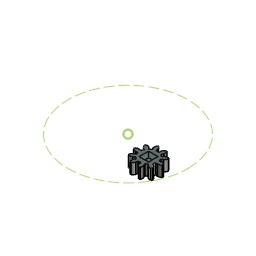
Electronics box (Autodesk Fusion 360 archive; units mm, degrees)
design "small gear"
description: Spur Gear; Module: 12.7; Num Teeth: 10; Pressure Angle: 20.0; Backlash: 0.00 mm
Autodesk Fusion 360 part; units mm, degrees
(part 1 of 4)
sketch "Sketch1" plane through (0, 0, 0) normal (0, 0, 1) x (1, 0, 0) in component "Spur Gear (10 teeth)"
  circle A0 centre (0, 0) radius 48.2092
  circle A1 centre (0, 0) radius 6.35
extrude "Extrude1" add sketch "Sketch1" along normal blind 12.7 in component "Spur Gear (10 teeth)"
sketch "Sketch2" plane through (0, 0, 0) normal (0, 0, 1) x (1, 0, 0) in component "Spur Gear (10 teeth)"
  spline S0 degree 5 poles (58.7902, -10.2119) (58.8398, -10.2205) (58.9391, -10.2359) (59.0886, -10.2539) (59.2889, -10.2679) (59.5405, -10.2721) (59.7929, -10.2667) (60.0458, -10.2556) (60.2991, -10.2415) (60.5524, -10.2252) (60.8059, -10.2064) (61.0595, -10.1843) (61.3132, -10.158) (61.5672, -10.1267) (61.8213, -10.0907) (62.0755, -10.0504) (62.3297, -10.0065) (62.5839, -9.9595) (62.838, -9.9098) (63.092, -9.8574) (63.3459, -9.8024) (63.5998, -9.7445) (63.8535, -9.6836) (64.107, -9.6197) (64.3605, -9.5529) (64.6138, -9.4832) (64.8669, -9.4108) (65.1198, -9.3359) (65.3724, -9.2586) (65.6249, -9.1787) (65.8771, -9.0965) (66.129, -9.0118) (66.3807, -8.9247) (66.6321, -8.8352) (66.8832, -8.7433) (67.134, -8.649) (67.3844, -8.5525) (67.6346, -8.4537) (67.8844, -8.3527) (68.1338, -8.2495) (68.3829, -8.1441) (68.6317, -8.0366) (68.88, -7.9269) (69.128, -7.8151) (69.3755, -7.7012) (69.6227, -7.5852) (69.8694, -7.4672) (70.1157, -7.3471) (70.3615, -7.2251) (70.6069, -7.101) (70.8519, -6.9749) (71.0964, -6.8469) (71.3404, -6.7169) (71.5839, -6.5851) (71.827, -6.4512) (72.0695, -6.3155) (72.3115, -6.1779) (72.5531, -6.0384) (72.7941, -5.8971) (73.0345, -5.7539) (73.2744, -5.6089) (73.5138, -5.4621) (73.7527, -5.3135) (73.9909, -5.1631) (74.2286, -5.0109) (74.4657, -4.857) (74.7023, -4.7013) (74.9382, -4.5438) (75.1735, -4.3847) (75.4083, -4.2238) (75.6424, -4.0612) (75.8292, -3.9298) (75.969, -3.8304) (76.0621, -3.7639) (76.1086, -3.7305) knots 0 0 0 0 0 0 0.01428571 0.02857143 0.04285714 0.05714286 0.07142857 0.08571429 0.1 0.11428571 0.12857143 0.14285714 0.15714286 0.17142857 0.18571429 0.2 0.21428571 0.22857143 0.24285714 0.25714286 0.27142857 0.28571429 0.3 0.31428571 0.32857143 0.34285714 0.35714286 0.37142857 0.38571429 0.4 0.41428571 0.42857143 0.44285714 0.45714286 0.47142857 0.48571429 0.5 0.51428571 0.52857143 0.54285714 0.55714286 0.57142857 0.58571429 0.6 0.61428571 0.62857143 0.64285714 0.65714286 0.67142857 0.68571429 0.7 0.71428571 0.72857143 0.74285714 0.75714286 0.77142857 0.78571429 0.8 0.81428571 0.82857143 0.84285714 0.85714286 0.87142857 0.88571429 0.9 0.91428571 0.92857143 0.94285714 0.95714286 0.97142857 0.98571429 1 1 1 1 1 1
  spline S1 degree 5 poles (58.7902, 10.2119) (58.8398, 10.2205) (58.9391, 10.2359) (59.0886, 10.2539) (59.2889, 10.2679) (59.5405, 10.2721) (59.7929, 10.2667) (60.0458, 10.2556) (60.2991, 10.2415) (60.5524, 10.2252) (60.8059, 10.2064) (61.0595, 10.1843) (61.3132, 10.158) (61.5672, 10.1267) (61.8213, 10.0907) (62.0755, 10.0504) (62.3297, 10.0065) (62.5839, 9.9595) (62.838, 9.9098) (63.092, 9.8574) (63.3459, 9.8024) (63.5998, 9.7445) (63.8535, 9.6836) (64.107, 9.6197) (64.3605, 9.5529) (64.6138, 9.4832) (64.8669, 9.4108) (65.1198, 9.3359) (65.3724, 9.2586) (65.6249, 9.1787) (65.8771, 9.0965) (66.129, 9.0118) (66.3807, 8.9247) (66.6321, 8.8352) (66.8832, 8.7433) (67.134, 8.649) (67.3844, 8.5525) (67.6346, 8.4537) (67.8844, 8.3527) (68.1338, 8.2495) (68.3829, 8.1441) (68.6317, 8.0366) (68.88, 7.9269) (69.128, 7.8151) (69.3755, 7.7012) (69.6227, 7.5852) (69.8694, 7.4672) (70.1157, 7.3471) (70.3615, 7.2251) (70.6069, 7.101) (70.8519, 6.9749) (71.0964, 6.8469) (71.3404, 6.7169) (71.5839, 6.5851) (71.827, 6.4512) (72.0695, 6.3155) (72.3115, 6.1779) (72.5531, 6.0384) (72.7941, 5.8971) (73.0345, 5.7539) (73.2744, 5.6089) (73.5138, 5.4621) (73.7527, 5.3135) (73.9909, 5.1631) (74.2286, 5.0109) (74.4657, 4.857) (74.7023, 4.7013) (74.9382, 4.5438) (75.1735, 4.3847) (75.4083, 4.2238) (75.6424, 4.0612) (75.8292, 3.9298) (75.969, 3.8304) (76.0621, 3.7639) (76.1086, 3.7305) knots 0 0 0 0 0 0 0.01428571 0.02857143 0.04285714 0.05714286 0.07142857 0.08571429 0.1 0.11428571 0.12857143 0.14285714 0.15714286 0.17142857 0.18571429 0.2 0.21428571 0.22857143 0.24285714 0.25714286 0.27142857 0.28571429 0.3 0.31428571 0.32857143 0.34285714 0.35714286 0.37142857 0.38571429 0.4 0.41428571 0.42857143 0.44285714 0.45714286 0.47142857 0.48571429 0.5 0.51428571 0.52857143 0.54285714 0.55714286 0.57142857 0.58571429 0.6 0.61428571 0.62857143 0.64285714 0.65714286 0.67142857 0.68571429 0.7 0.71428571 0.72857143 0.74285714 0.75714286 0.77142857 0.78571429 0.8 0.81428571 0.82857143 0.84285714 0.85714286 0.87142857 0.88571429 0.9 0.91428571 0.92857143 0.94285714 0.95714286 0.97142857 0.98571429 1 1 1 1 1 1
  arc A0 (76.1086, -3.7305) -> (76.1086, 3.7305) centre (0, 0) ccw
  line L0 (47.4881, -8.2504) -> (58.7902, -10.2119)
  line L1 (47.4881, 8.2504) -> (58.7902, 10.2119)
  line L2 (47.4881, -8.2504) -> (47.4881, 8.2504)
  point P0 (59.9803, -10.2579)
  point P1 (61.1925, -10.1699)
  point P2 (62.4182, -9.9897)
  point P3 (63.6537, -9.7311)
  point P4 (64.8964, -9.4016)
  point P5 (66.1443, -9.006)
  point P6 (67.3954, -8.5476)
  point P7 (68.648, -8.0288)
  point P8 (69.9005, -7.4516)
  point P9 (71.1514, -6.8172)
  point P10 (72.3992, -6.127)
  point P11 (73.6422, -5.382)
  point P12 (74.8792, -4.5829)
  point P13 (59.9803, 10.2579)
  point P14 (61.1925, 10.1699)
  point P15 (62.4182, 9.9897)
  point P16 (63.6537, 9.7311)
  point P17 (64.8964, 9.4016)
  point P18 (66.1443, 9.006)
  point P19 (67.3954, 8.5476)
  point P20 (68.648, 8.0288)
  point P21 (69.9005, 7.4516)
  point P22 (71.1514, 6.8172)
  point P23 (72.3992, 6.127)
  point P24 (73.6422, 5.382)
  point P25 (74.8792, 4.5829)
extrude "Extrude2" add sketch "Sketch2" along normal blind 12.7 in component "Spur Gear (10 teeth)"
fillet "Fillet1" radius 1.5875 2 edges at (47.4977, -8.2521, 6.35) (47.4977, 8.2521, 6.35) in component "Spur Gear (10 teeth)"
pattern_circular "C-Pattern1" count 10 over 360 about axis through (0, 0, 0) along (0, 0, 1) of "Extrude2", "Fillet1" in component "Spur Gear (10 teeth)"
sketch "Sketch3" plane through (0, 0, 0) normal (0, 0, 1) x (1, 0, 0) in component "Spur Gear (10 teeth)"
  circle A0 centre (0, 0) radius 63.5 construction
scale "Scale1" factor 0.2 about (53.5646, -26.2944, 0) bodies 1 in component "Spur Gear (10 teeth)"
extrude "Extrude3" add 1 faces at (37.4307, -25.0246, 2.54) along direction (0, 0, 1) blind 8.73 in component "Spur Gear (10 teeth)"
sketch "Sketch2 (2)" plane through (0, 0, 11.27) normal (0, 0, 1) x (-1, 0, 0)
  arc A0 (-51.6381, 25.006) -> (-52.2938, 22.9879) centre (-42.8517, 21.0355) ccw
  arc A1 (-52.659, 22.7394) -> (-52.2938, 22.9879) centre (-52.6047, 23.0522) ccw
  line L0 (-52.659, 22.7394) -> (-54.6097, 23.0779)
  spline S0 degree 5 poles (-54.6097, 23.0779) (-54.6197, 23.0796) (-54.6395, 23.0827) (-54.6694, 23.0863) (-54.7095, 23.0891) (-54.7598, 23.09) (-54.8103, 23.0889) (-54.8609, 23.0867) (-54.9115, 23.0838) (-54.9622, 23.0806) (-55.0129, 23.0768) (-55.0636, 23.0724) (-55.1143, 23.0671) (-55.1651, 23.0609) (-55.216, 23.0537) (-55.2668, 23.0456) (-55.3176, 23.0368) (-55.3685, 23.0274) (-55.4193, 23.0175) (-55.4701, 23.007) (-55.5209, 22.996) (-55.5717, 22.9844) (-55.6224, 22.9723) (-55.6731, 22.9595) (-55.7238, 22.9461) (-55.7745, 22.9322) (-55.8251, 22.9177) (-55.8757, 22.9027) (-55.9262, 22.8873) (-55.9767, 22.8713) (-56.0271, 22.8548) (-56.0775, 22.8379) (-56.1278, 22.8205) (-56.1781, 22.8026) (-56.2283, 22.7842) (-56.2785, 22.7653) (-56.3286, 22.746) (-56.3786, 22.7263) (-56.4286, 22.7061) (-56.4785, 22.6854) (-56.5283, 22.6644) (-56.578, 22.6429) (-56.6277, 22.6209) (-56.6773, 22.5986) (-56.7268, 22.5758) (-56.7762, 22.5526) (-56.8256, 22.529) (-56.8748, 22.505) (-56.924, 22.4806) (-56.9731, 22.4557) (-57.0221, 22.4305) (-57.071, 22.4049) (-57.1198, 22.3789) (-57.1685, 22.3526) (-57.2171, 22.3258) (-57.2656, 22.2987) (-57.314, 22.2711) (-57.3623, 22.2432) (-57.4105, 22.215) (-57.4586, 22.1863) (-57.5066, 22.1573) (-57.5545, 22.128) (-57.6022, 22.0982) (-57.6499, 22.0682) (-57.6974, 22.0377) (-57.7448, 22.0069) (-57.7922, 21.9758) (-57.8393, 21.9443) (-57.8864, 21.9125) (-57.9334, 21.8803) (-57.9802, 21.8478) (-58.0175, 21.8215) (-58.0455, 21.8016) (-58.0641, 21.7883) (-58.0734, 21.7816) knots 0 0 0 0 0 0 0.01428571 0.02857143 0.04285714 0.05714286 0.07142857 0.08571429 0.1 0.11428571 0.12857143 0.14285714 0.15714286 0.17142857 0.18571429 0.2 0.21428571 0.22857143 0.24285714 0.25714286 0.27142857 0.28571429 0.3 0.31428571 0.32857143 0.34285714 0.35714286 0.37142857 0.38571429 0.4 0.41428571 0.42857143 0.44285714 0.45714286 0.47142857 0.48571429 0.5 0.51428571 0.52857143 0.54285714 0.55714286 0.57142857 0.58571429 0.6 0.61428571 0.62857143 0.64285714 0.65714286 0.67142857 0.68571429 0.7 0.71428571 0.72857143 0.74285714 0.75714286 0.77142857 0.78571429 0.8 0.81428571 0.82857143 0.84285714 0.85714286 0.87142857 0.88571429 0.9 0.91428571 0.92857143 0.94285714 0.95714286 0.97142857 0.98571429 1 1 1 1 1 1
  arc A2 (-58.0734, 21.7816) -> (-58.0734, 20.2895) centre (-42.8517, 21.0355) ccw
  spline S1 degree 5 poles (-58.0734, 20.2895) (-58.0641, 20.2828) (-58.0455, 20.2695) (-58.0175, 20.2496) (-57.9802, 20.2233) (-57.9334, 20.1908) (-57.8864, 20.1586) (-57.8393, 20.1268) (-57.7922, 20.0953) (-57.7448, 20.0642) (-57.6974, 20.0334) (-57.6499, 20.0029) (-57.6022, 19.9728) (-57.5545, 19.9431) (-57.5066, 19.9138) (-57.4586, 19.8848) (-57.4105, 19.8561) (-57.3623, 19.8279) (-57.314, 19.8) (-57.2656, 19.7724) (-57.2171, 19.7453) (-57.1685, 19.7185) (-57.1198, 19.6922) (-57.071, 19.6662) (-57.0221, 19.6406) (-56.9731, 19.6154) (-56.924, 19.5905) (-56.8748, 19.5661) (-56.8256, 19.5421) (-56.7762, 19.5185) (-56.7268, 19.4953) (-56.6773, 19.4725) (-56.6277, 19.4502) (-56.578, 19.4282) (-56.5283, 19.4067) (-56.4785, 19.3857) (-56.4286, 19.365) (-56.3786, 19.3448) (-56.3286, 19.3251) (-56.2785, 19.3057) (-56.2283, 19.2869) (-56.1781, 19.2685) (-56.1278, 19.2506) (-56.0775, 19.2332) (-56.0271, 19.2162) (-55.9767, 19.1998) (-55.9262, 19.1838) (-55.8757, 19.1684) (-55.8251, 19.1534) (-55.7745, 19.1389) (-55.7238, 19.125) (-55.6731, 19.1116) (-55.6224, 19.0988) (-55.5717, 19.0866) (-55.5209, 19.0751) (-55.4701, 19.0641) (-55.4193, 19.0536) (-55.3685, 19.0437) (-55.3176, 19.0343) (-55.2668, 19.0255) (-55.216, 19.0174) (-55.1651, 19.0102) (-55.1143, 19.004) (-55.0636, 18.9987) (-55.0129, 18.9943) (-54.9622, 18.9905) (-54.9115, 18.9873) (-54.8609, 18.9844) (-54.8103, 18.9822) (-54.7598, 18.9811) (-54.7095, 18.982) (-54.6694, 18.9848) (-54.6395, 18.9884) (-54.6197, 18.9915) (-54.6097, 18.9932) knots -1 -1 -1 -1 -1 -1 -0.98571429 -0.97142857 -0.95714286 -0.94285714 -0.92857143 -0.91428571 -0.9 -0.88571429 -0.87142857 -0.85714286 -0.84285714 -0.82857143 -0.81428571 -0.8 -0.78571429 -0.77142857 -0.75714286 -0.74285714 -0.72857143 -0.71428571 -0.7 -0.68571429 -0.67142857 -0.65714286 -0.64285714 -0.62857143 -0.61428571 -0.6 -0.58571429 -0.57142857 -0.55714286 -0.54285714 -0.52857143 -0.51428571 -0.5 -0.48571429 -0.47142857 -0.45714286 -0.44285714 -0.42857143 -0.41428571 -0.4 -0.38571429 -0.37142857 -0.35714286 -0.34285714 -0.32857143 -0.31428571 -0.3 -0.28571429 -0.27142857 -0.25714286 -0.24285714 -0.22857143 -0.21428571 -0.2 -0.18571429 -0.17142857 -0.15714286 -0.14285714 -0.12857143 -0.11428571 -0.1 -0.08571429 -0.07142857 -0.05714286 -0.04285714 -0.02857143 -0.01428571 0 0 0 0 0 0
  line L1 (-54.6097, 18.9932) -> (-52.659, 19.3317)
  arc A3 (-52.2938, 19.0832) -> (-52.659, 19.3317) centre (-52.6047, 19.0189) ccw
  arc A4 (-52.2938, 19.0832) -> (-51.6381, 17.0651) centre (-42.8517, 21.0355) ccw
  arc A5 (-51.7875, 16.6494) -> (-51.6381, 17.0651) centre (-51.9274, 16.9344) ccw
  line L2 (-51.7875, 16.6494) -> (-53.5646, 15.7767)
  spline S2 degree 5 poles (-53.5646, 15.7767) (-53.5737, 15.7722) (-53.5916, 15.763) (-53.6179, 15.7484) (-53.6519, 15.7271) (-53.6931, 15.6982) (-53.7333, 15.6677) (-53.7729, 15.6361) (-53.8123, 15.6041) (-53.8513, 15.5716) (-53.8901, 15.5388) (-53.9286, 15.5054) (-53.9665, 15.4713) (-54.0039, 15.4364) (-54.0408, 15.4007) (-54.0772, 15.3643) (-54.1132, 15.3273) (-54.1488, 15.2898) (-54.1841, 15.2519) (-54.219, 15.2136) (-54.2536, 15.1748) (-54.2879, 15.1356) (-54.3218, 15.096) (-54.3553, 15.0558) (-54.3885, 15.0152) (-54.4212, 14.9742) (-54.4537, 14.9327) (-54.4858, 14.8908) (-54.5176, 14.8486) (-54.5491, 14.806) (-54.5802, 14.7631) (-54.611, 14.7198) (-54.6415, 14.6761) (-54.6716, 14.632) (-54.7015, 14.5876) (-54.731, 14.5429) (-54.7601, 14.4978) (-54.789, 14.4525) (-54.8175, 14.4067) (-54.8458, 14.3607) (-54.8737, 14.3144) (-54.9013, 14.2678) (-54.9286, 14.2208) (-54.9556, 14.1736) (-54.9822, 14.126) (-55.0086, 14.0782) (-55.0346, 14.0301) (-55.0604, 13.9817) (-55.0858, 13.9331) (-55.1109, 13.8842) (-55.1357, 13.835) (-55.1602, 13.7855) (-55.1844, 13.7358) (-55.2083, 13.6858) (-55.2319, 13.6356) (-55.2552, 13.5851) (-55.2782, 13.5344) (-55.3009, 13.4835) (-55.3233, 13.4323) (-55.3454, 13.3808) (-55.3671, 13.3292) (-55.3886, 13.2773) (-55.4098, 13.2251) (-55.4306, 13.1728) (-55.4512, 13.1202) (-55.4715, 13.0674) (-55.4914, 13.0144) (-55.5111, 12.9612) (-55.5305, 12.9078) (-55.5495, 12.8542) (-55.5683, 12.8004) (-55.5831, 12.7571) (-55.594, 12.7246) (-55.6013, 12.7029) (-55.6049, 12.692) knots 0 0 0 0 0 0 0.01428571 0.02857143 0.04285714 0.05714286 0.07142857 0.08571429 0.1 0.11428571 0.12857143 0.14285714 0.15714286 0.17142857 0.18571429 0.2 0.21428571 0.22857143 0.24285714 0.25714286 0.27142857 0.28571429 0.3 0.31428571 0.32857143 0.34285714 0.35714286 0.37142857 0.38571429 0.4 0.41428571 0.42857143 0.44285714 0.45714286 0.47142857 0.48571429 0.5 0.51428571 0.52857143 0.54285714 0.55714286 0.57142857 0.58571429 0.6 0.61428571 0.62857143 0.64285714 0.65714286 0.67142857 0.68571429 0.7 0.71428571 0.72857143 0.74285714 0.75714286 0.77142857 0.78571429 0.8 0.81428571 0.82857143 0.84285714 0.85714286 0.87142857 0.88571429 0.9 0.91428571 0.92857143 0.94285714 0.95714286 0.97142857 0.98571429 1 1 1 1 1 1
  arc A6 (-55.6049, 12.692) -> (-54.7278, 11.4848) centre (-42.8517, 21.0355) ccw
  spline S3 degree 5 poles (-54.7278, 11.4848) (-54.7163, 11.4849) (-54.6935, 11.4851) (-54.6591, 11.4854) (-54.6135, 11.4861) (-54.5565, 11.4874) (-54.4996, 11.4889) (-54.4428, 11.4908) (-54.3861, 11.4931) (-54.3295, 11.4957) (-54.2731, 11.4987) (-54.2167, 11.502) (-54.1605, 11.5057) (-54.1044, 11.5097) (-54.0484, 11.5141) (-53.9925, 11.5188) (-53.9368, 11.5239) (-53.8812, 11.5294) (-53.8257, 11.5352) (-53.7704, 11.5414) (-53.7152, 11.5479) (-53.6601, 11.5549) (-53.6052, 11.5622) (-53.5504, 11.5698) (-53.4958, 11.5778) (-53.4414, 11.5862) (-53.3871, 11.595) (-53.3329, 11.6042) (-53.279, 11.6137) (-53.2252, 11.6236) (-53.1716, 11.6339) (-53.1181, 11.6446) (-53.0649, 11.6556) (-53.0118, 11.6671) (-52.9589, 11.6789) (-52.9062, 11.6911) (-52.8537, 11.7038) (-52.8014, 11.7168) (-52.7493, 11.7302) (-52.6975, 11.744) (-52.6458, 11.7583) (-52.5944, 11.7729) (-52.5432, 11.788) (-52.4922, 11.8035) (-52.4415, 11.8194) (-52.391, 11.8357) (-52.3408, 11.8525) (-52.2908, 11.8697) (-52.2411, 11.8873) (-52.1916, 11.9053) (-52.1424, 11.9238) (-52.0936, 11.9428) (-52.045, 11.9623) (-51.9968, 11.9823) (-51.9489, 12.0027) (-51.9014, 12.0237) (-51.8541, 12.0451) (-51.8072, 12.0669) (-51.7605, 12.0892) (-51.7142, 12.1119) (-51.6684, 12.1353) (-51.623, 12.1594) (-51.5783, 12.1842) (-51.5341, 12.2097) (-51.4905, 12.236) (-51.4472, 12.2627) (-51.4043, 12.2899) (-51.3617, 12.3173) (-51.3195, 12.3453) (-51.278, 12.3741) (-51.2378, 12.4043) (-51.207, 12.4301) (-51.1849, 12.4506) (-51.1707, 12.4648) (-51.1637, 12.472) knots -1 -1 -1 -1 -1 -1 -0.98571429 -0.97142857 -0.95714286 -0.94285714 -0.92857143 -0.91428571 -0.9 -0.88571429 -0.87142857 -0.85714286 -0.84285714 -0.82857143 -0.81428571 -0.8 -0.78571429 -0.77142857 -0.75714286 -0.74285714 -0.72857143 -0.71428571 -0.7 -0.68571429 -0.67142857 -0.65714286 -0.64285714 -0.62857143 -0.61428571 -0.6 -0.58571429 -0.57142857 -0.55714286 -0.54285714 -0.52857143 -0.51428571 -0.5 -0.48571429 -0.47142857 -0.45714286 -0.44285714 -0.42857143 -0.41428571 -0.4 -0.38571429 -0.37142857 -0.35714286 -0.34285714 -0.32857143 -0.31428571 -0.3 -0.28571429 -0.27142857 -0.25714286 -0.24285714 -0.22857143 -0.21428571 -0.2 -0.18571429 -0.17142857 -0.15714286 -0.14285714 -0.12857143 -0.11428571 -0.1 -0.08571429 -0.07142857 -0.05714286 -0.04285714 -0.02857143 -0.01428571 0 0 0 0 0 0
  line L3 (-51.1637, 12.472) -> (-49.7845, 13.8925)
  arc A7 (-49.343, 13.9061) -> (-49.7845, 13.8925) centre (-49.5567, 13.6714) ccw
  arc A8 (-49.343, 13.9061) -> (-47.6263, 12.6589) centre (-42.8517, 21.0355) ccw
  arc A9 (-47.5028, 12.2347) -> (-47.6263, 12.6589) centre (-47.7835, 12.383) ccw
  line L4 (-47.5028, 12.2347) -> (-48.4275, 10.4841)
  spline S4 degree 5 poles (-48.4275, 10.4841) (-48.4322, 10.4752) (-48.4413, 10.4573) (-48.454, 10.4299) (-48.469, 10.3927) (-48.4854, 10.3451) (-48.4999, 10.2968) (-48.5135, 10.248) (-48.5264, 10.1989) (-48.539, 10.1497) (-48.5511, 10.1004) (-48.5626, 10.0508) (-48.5732, 10.0009) (-48.583, 9.9506) (-48.5918, 9.9001) (-48.5999, 9.8492) (-48.6072, 9.7982) (-48.614, 9.7469) (-48.6202, 9.6955) (-48.626, 9.644) (-48.6312, 9.5923) (-48.6359, 9.5404) (-48.64, 9.4884) (-48.6435, 9.4362) (-48.6465, 9.3839) (-48.6489, 9.3314) (-48.6507, 9.2788) (-48.6521, 9.226) (-48.653, 9.1732) (-48.6534, 9.1202) (-48.6534, 9.0672) (-48.6528, 9.014) (-48.6518, 8.9608) (-48.6503, 8.9074) (-48.6484, 8.854) (-48.6459, 8.8004) (-48.6431, 8.7468) (-48.6397, 8.6932) (-48.636, 8.6394) (-48.6317, 8.5856) (-48.6271, 8.5317) (-48.622, 8.4777) (-48.6165, 8.4237) (-48.6106, 8.3696) (-48.6042, 8.3155) (-48.5974, 8.2613) (-48.5902, 8.2071) (-48.5826, 8.1528) (-48.5746, 8.0985) (-48.5661, 8.0442) (-48.5573, 7.9898) (-48.5481, 7.9354) (-48.5384, 7.8809) (-48.5284, 7.8265) (-48.5179, 7.772) (-48.5071, 7.7174) (-48.4959, 7.6629) (-48.4843, 7.6083) (-48.4723, 7.5538) (-48.4599, 7.4992) (-48.4472, 7.4446) (-48.4341, 7.39) (-48.4206, 7.3354) (-48.4067, 7.2807) (-48.3924, 7.2261) (-48.3778, 7.1715) (-48.3628, 7.1169) (-48.3474, 7.0623) (-48.3317, 7.0077) (-48.3156, 6.9531) (-48.2991, 6.8985) (-48.2857, 6.8549) (-48.2754, 6.8221) (-48.2685, 6.8003) (-48.2651, 6.7894) knots 0 0 0 0 0 0 0.01428571 0.02857143 0.04285714 0.05714286 0.07142857 0.08571429 0.1 0.11428571 0.12857143 0.14285714 0.15714286 0.17142857 0.18571429 0.2 0.21428571 0.22857143 0.24285714 0.25714286 0.27142857 0.28571429 0.3 0.31428571 0.32857143 0.34285714 0.35714286 0.37142857 0.38571429 0.4 0.41428571 0.42857143 0.44285714 0.45714286 0.47142857 0.48571429 0.5 0.51428571 0.52857143 0.54285714 0.55714286 0.57142857 0.58571429 0.6 0.61428571 0.62857143 0.64285714 0.65714286 0.67142857 0.68571429 0.7 0.71428571 0.72857143 0.74285714 0.75714286 0.77142857 0.78571429 0.8 0.81428571 0.82857143 0.84285714 0.85714286 0.87142857 0.88571429 0.9 0.91428571 0.92857143 0.94285714 0.95714286 0.97142857 0.98571429 1 1 1 1 1 1
  arc A10 (-48.2651, 6.7894) -> (-46.8459, 6.3283) centre (-42.8517, 21.0355) ccw
  spline S5 degree 5 poles (-46.8459, 6.3283) (-46.8367, 6.3351) (-46.8183, 6.3486) (-46.7907, 6.3691) (-46.7542, 6.3965) (-46.7088, 6.431) (-46.6637, 6.4657) (-46.6188, 6.5006) (-46.5743, 6.5358) (-46.5301, 6.5711) (-46.4861, 6.6067) (-46.4425, 6.6425) (-46.3992, 6.6786) (-46.3561, 6.7148) (-46.3134, 6.7513) (-46.271, 6.7879) (-46.2289, 6.8248) (-46.1871, 6.8619) (-46.1457, 6.8993) (-46.1046, 6.9368) (-46.0638, 6.9745) (-46.0233, 7.0125) (-45.9831, 7.0507) (-45.9433, 7.089) (-45.9039, 7.1276) (-45.8648, 7.1664) (-45.826, 7.2055) (-45.7876, 7.2447) (-45.7495, 7.2841) (-45.7118, 7.3237) (-45.6745, 7.3636) (-45.6375, 7.4036) (-45.6009, 7.4439) (-45.5647, 7.4843) (-45.5289, 7.525) (-45.4935, 7.5659) (-45.4584, 7.6069) (-45.4238, 7.6482) (-45.3895, 7.6897) (-45.3557, 7.7314) (-45.3222, 7.7733) (-45.2892, 7.8153) (-45.2567, 7.8576) (-45.2245, 7.9001) (-45.1929, 7.9428) (-45.1616, 7.9857) (-45.1309, 8.0288) (-45.1005, 8.072) (-45.0706, 8.1155) (-45.0412, 8.1592) (-45.0123, 8.2031) (-44.984, 8.2471) (-44.9561, 8.2914) (-44.9289, 8.3359) (-44.9022, 8.3806) (-44.876, 8.4255) (-44.8504, 8.4706) (-44.8252, 8.5159) (-44.8005, 8.5613) (-44.7765, 8.6069) (-44.7531, 8.6528) (-44.7305, 8.6989) (-44.7089, 8.7453) (-44.6882, 8.7919) (-44.6683, 8.8388) (-44.6491, 8.8858) (-44.6303, 8.933) (-44.612, 8.9803) (-44.5943, 9.0277) (-44.5776, 9.0754) (-44.5629, 9.1235) (-44.5532, 9.1625) (-44.5473, 9.192) (-44.5442, 9.2119) (-44.5427, 9.2219) knots -1 -1 -1 -1 -1 -1 -0.98571429 -0.97142857 -0.95714286 -0.94285714 -0.92857143 -0.91428571 -0.9 -0.88571429 -0.87142857 -0.85714286 -0.84285714 -0.82857143 -0.81428571 -0.8 -0.78571429 -0.77142857 -0.75714286 -0.74285714 -0.72857143 -0.71428571 -0.7 -0.68571429 -0.67142857 -0.65714286 -0.64285714 -0.62857143 -0.61428571 -0.6 -0.58571429 -0.57142857 -0.55714286 -0.54285714 -0.52857143 -0.51428571 -0.5 -0.48571429 -0.47142857 -0.45714286 -0.44285714 -0.42857143 -0.41428571 -0.4 -0.38571429 -0.37142857 -0.35714286 -0.34285714 -0.32857143 -0.31428571 -0.3 -0.28571429 -0.27142857 -0.25714286 -0.24285714 -0.22857143 -0.21428571 -0.2 -0.18571429 -0.17142857 -0.15714286 -0.14285714 -0.12857143 -0.11428571 -0.1 -0.08571429 -0.07142857 -0.05714286 -0.04285714 -0.02857143 -0.01428571 0 0 0 0 0 0
  line L5 (-44.5427, 9.2219) -> (-44.2619, 11.1817)
  arc A11 (-43.9127, 11.4523) -> (-44.2619, 11.1817) centre (-43.9476, 11.1367) ccw
  arc A12 (-43.9127, 11.4523) -> (-41.7907, 11.4523) centre (-42.8517, 21.0355) ccw
  arc A13 (-41.4415, 11.1817) -> (-41.7907, 11.4523) centre (-41.7558, 11.1367) ccw
  line L6 (-41.4415, 11.1817) -> (-41.1607, 9.2219)
  spline S6 degree 5 poles (-41.1607, 9.2219) (-41.1592, 9.2119) (-41.1561, 9.192) (-41.1502, 9.1625) (-41.1405, 9.1235) (-41.1258, 9.0754) (-41.1091, 9.0277) (-41.0914, 8.9803) (-41.0731, 8.933) (-41.0543, 8.8858) (-41.0351, 8.8388) (-41.0152, 8.7919) (-40.9945, 8.7453) (-40.9729, 8.6989) (-40.9503, 8.6528) (-40.9269, 8.6069) (-40.9029, 8.5613) (-40.8782, 8.5159) (-40.853, 8.4706) (-40.8274, 8.4255) (-40.8012, 8.3806) (-40.7745, 8.3359) (-40.7473, 8.2914) (-40.7194, 8.2471) (-40.6911, 8.2031) (-40.6622, 8.1592) (-40.6328, 8.1155) (-40.6029, 8.072) (-40.5725, 8.0288) (-40.5418, 7.9857) (-40.5105, 7.9428) (-40.4789, 7.9001) (-40.4467, 7.8576) (-40.4142, 7.8153) (-40.3812, 7.7733) (-40.3477, 7.7314) (-40.3139, 7.6897) (-40.2796, 7.6482) (-40.245, 7.6069) (-40.2099, 7.5659) (-40.1745, 7.525) (-40.1387, 7.4843) (-40.1025, 7.4439) (-40.0659, 7.4036) (-40.0289, 7.3636) (-39.9916, 7.3237) (-39.9539, 7.2841) (-39.9158, 7.2447) (-39.8774, 7.2055) (-39.8386, 7.1664) (-39.7995, 7.1276) (-39.7601, 7.089) (-39.7203, 7.0507) (-39.6801, 7.0125) (-39.6396, 6.9745) (-39.5988, 6.9368) (-39.5577, 6.8993) (-39.5163, 6.8619) (-39.4745, 6.8248) (-39.4324, 6.7879) (-39.39, 6.7513) (-39.3473, 6.7148) (-39.3042, 6.6786) (-39.2609, 6.6425) (-39.2173, 6.6067) (-39.1733, 6.5711) (-39.1291, 6.5358) (-39.0846, 6.5006) (-39.0397, 6.4657) (-38.9946, 6.431) (-38.9492, 6.3965) (-38.9127, 6.3691) (-38.8851, 6.3486) (-38.8667, 6.3351) (-38.8575, 6.3283) knots 0 0 0 0 0 0 0.01428571 0.02857143 0.04285714 0.05714286 0.07142857 0.08571429 0.1 0.11428571 0.12857143 0.14285714 0.15714286 0.17142857 0.18571429 0.2 0.21428571 0.22857143 0.24285714 0.25714286 0.27142857 0.28571429 0.3 0.31428571 0.32857143 0.34285714 0.35714286 0.37142857 0.38571429 0.4 0.41428571 0.42857143 0.44285714 0.45714286 0.47142857 0.48571429 0.5 0.51428571 0.52857143 0.54285714 0.55714286 0.57142857 0.58571429 0.6 0.61428571 0.62857143 0.64285714 0.65714286 0.67142857 0.68571429 0.7 0.71428571 0.72857143 0.74285714 0.75714286 0.77142857 0.78571429 0.8 0.81428571 0.82857143 0.84285714 0.85714286 0.87142857 0.88571429 0.9 0.91428571 0.92857143 0.94285714 0.95714286 0.97142857 0.98571429 1 1 1 1 1 1
  arc A14 (-38.8575, 6.3283) -> (-37.4383, 6.7894) centre (-42.8517, 21.0355) ccw
  spline S7 degree 5 poles (-37.4383, 6.7894) (-37.4349, 6.8003) (-37.428, 6.8221) (-37.4177, 6.8549) (-37.4043, 6.8985) (-37.3878, 6.9531) (-37.3717, 7.0077) (-37.356, 7.0623) (-37.3406, 7.1169) (-37.3256, 7.1715) (-37.311, 7.2261) (-37.2967, 7.2807) (-37.2828, 7.3354) (-37.2693, 7.39) (-37.2562, 7.4446) (-37.2435, 7.4992) (-37.2311, 7.5538) (-37.2191, 7.6083) (-37.2075, 7.6629) (-37.1963, 7.7174) (-37.1855, 7.772) (-37.175, 7.8265) (-37.165, 7.8809) (-37.1553, 7.9354) (-37.1461, 7.9898) (-37.1373, 8.0442) (-37.1288, 8.0985) (-37.1208, 8.1528) (-37.1132, 8.2071) (-37.106, 8.2613) (-37.0992, 8.3155) (-37.0928, 8.3696) (-37.0869, 8.4237) (-37.0814, 8.4777) (-37.0763, 8.5317) (-37.0717, 8.5856) (-37.0674, 8.6394) (-37.0637, 8.6932) (-37.0603, 8.7468) (-37.0575, 8.8004) (-37.055, 8.854) (-37.0531, 8.9074) (-37.0516, 8.9608) (-37.0506, 9.014) (-37.05, 9.0672) (-37.05, 9.1202) (-37.0504, 9.1732) (-37.0513, 9.226) (-37.0527, 9.2788) (-37.0545, 9.3314) (-37.0569, 9.3839) (-37.0599, 9.4362) (-37.0634, 9.4884) (-37.0675, 9.5404) (-37.0722, 9.5923) (-37.0774, 9.644) (-37.0832, 9.6955) (-37.0894, 9.7469) (-37.0962, 9.7982) (-37.1035, 9.8492) (-37.1116, 9.9001) (-37.1204, 9.9506) (-37.1302, 10.0009) (-37.1408, 10.0508) (-37.1523, 10.1004) (-37.1644, 10.1497) (-37.177, 10.1989) (-37.1899, 10.248) (-37.2035, 10.2968) (-37.218, 10.3451) (-37.2344, 10.3927) (-37.2494, 10.4299) (-37.2621, 10.4573) (-37.2712, 10.4752) (-37.2759, 10.4841) knots -1 -1 -1 -1 -1 -1 -0.98571429 -0.97142857 -0.95714286 -0.94285714 -0.92857143 -0.91428571 -0.9 -0.88571429 -0.87142857 -0.85714286 -0.84285714 -0.82857143 -0.81428571 -0.8 -0.78571429 -0.77142857 -0.75714286 -0.74285714 -0.72857143 -0.71428571 -0.7 -0.68571429 -0.67142857 -0.65714286 -0.64285714 -0.62857143 -0.61428571 -0.6 -0.58571429 -0.57142857 -0.55714286 -0.54285714 -0.52857143 -0.51428571 -0.5 -0.48571429 -0.47142857 -0.45714286 -0.44285714 -0.42857143 -0.41428571 -0.4 -0.38571429 -0.37142857 -0.35714286 -0.34285714 -0.32857143 -0.31428571 -0.3 -0.28571429 -0.27142857 -0.25714286 -0.24285714 -0.22857143 -0.21428571 -0.2 -0.18571429 -0.17142857 -0.15714286 -0.14285714 -0.12857143 -0.11428571 -0.1 -0.08571429 -0.07142857 -0.05714286 -0.04285714 -0.02857143 -0.01428571 0 0 0 0 0 0
  line L7 (-37.2759, 10.4841) -> (-38.2006, 12.2347)
  arc A15 (-38.0771, 12.6589) -> (-38.2006, 12.2347) centre (-37.9199, 12.383) ccw
  arc A16 (-38.0771, 12.6589) -> (-36.3604, 13.9061) centre (-42.8517, 21.0355) ccw
  arc A17 (-35.9189, 13.8925) -> (-36.3604, 13.9061) centre (-36.1467, 13.6714) ccw
  line L8 (-35.9189, 13.8925) -> (-34.5397, 12.472)
  spline S8 degree 5 poles (-34.5397, 12.472) (-34.5327, 12.4648) (-34.5185, 12.4506) (-34.4964, 12.4301) (-34.4656, 12.4043) (-34.4254, 12.3741) (-34.3839, 12.3453) (-34.3417, 12.3173) (-34.2991, 12.2899) (-34.2562, 12.2627) (-34.2129, 12.236) (-34.1693, 12.2097) (-34.1252, 12.1842) (-34.0804, 12.1594) (-34.035, 12.1353) (-33.9892, 12.1119) (-33.9429, 12.0892) (-33.8962, 12.0669) (-33.8493, 12.0451) (-33.802, 12.0237) (-33.7545, 12.0027) (-33.7066, 11.9823) (-33.6584, 11.9623) (-33.6098, 11.9428) (-33.561, 11.9238) (-33.5118, 11.9053) (-33.4623, 11.8873) (-33.4126, 11.8697) (-33.3626, 11.8525) (-33.3124, 11.8357) (-33.2619, 11.8194) (-33.2112, 11.8035) (-33.1602, 11.788) (-33.109, 11.7729) (-33.0576, 11.7583) (-33.0059, 11.744) (-32.9541, 11.7302) (-32.902, 11.7168) (-32.8497, 11.7038) (-32.7972, 11.6911) (-32.7445, 11.6789) (-32.6916, 11.6671) (-32.6385, 11.6556) (-32.5853, 11.6446) (-32.5318, 11.6339) (-32.4782, 11.6236) (-32.4244, 11.6137) (-32.3705, 11.6042) (-32.3163, 11.595) (-32.262, 11.5862) (-32.2076, 11.5778) (-32.153, 11.5698) (-32.0982, 11.5622) (-32.0433, 11.5549) (-31.9882, 11.5479) (-31.933, 11.5414) (-31.8777, 11.5352) (-31.8222, 11.5294) (-31.7666, 11.5239) (-31.7109, 11.5188) (-31.655, 11.5141) (-31.599, 11.5097) (-31.5429, 11.5057) (-31.4867, 11.502) (-31.4303, 11.4987) (-31.3739, 11.4957) (-31.3173, 11.4931) (-31.2606, 11.4908) (-31.2038, 11.4889) (-31.1469, 11.4874) (-31.0899, 11.4861) (-31.0443, 11.4854) (-31.0099, 11.4851) (-30.9871, 11.4849) (-30.9756, 11.4848) knots 0 0 0 0 0 0 0.01428571 0.02857143 0.04285714 0.05714286 0.07142857 0.08571429 0.1 0.11428571 0.12857143 0.14285714 0.15714286 0.17142857 0.18571429 0.2 0.21428571 0.22857143 0.24285714 0.25714286 0.27142857 0.28571429 0.3 0.31428571 0.32857143 0.34285714 0.35714286 0.37142857 0.38571429 0.4 0.41428571 0.42857143 0.44285714 0.45714286 0.47142857 0.48571429 0.5 0.51428571 0.52857143 0.54285714 0.55714286 0.57142857 0.58571429 0.6 0.61428571 0.62857143 0.64285714 0.65714286 0.67142857 0.68571429 0.7 0.71428571 0.72857143 0.74285714 0.75714286 0.77142857 0.78571429 0.8 0.81428571 0.82857143 0.84285714 0.85714286 0.87142857 0.88571429 0.9 0.91428571 0.92857143 0.94285714 0.95714286 0.97142857 0.98571429 1 1 1 1 1 1
  arc A18 (-30.9756, 11.4848) -> (-30.0985, 12.692) centre (-42.8517, 21.0355) ccw
  spline S9 degree 5 poles (-30.0985, 12.692) (-30.1021, 12.7029) (-30.1094, 12.7246) (-30.1203, 12.7571) (-30.1351, 12.8004) (-30.1539, 12.8542) (-30.1729, 12.9078) (-30.1923, 12.9612) (-30.212, 13.0144) (-30.2319, 13.0674) (-30.2522, 13.1202) (-30.2728, 13.1728) (-30.2936, 13.2251) (-30.3148, 13.2773) (-30.3363, 13.3292) (-30.358, 13.3808) (-30.3801, 13.4323) (-30.4025, 13.4835) (-30.4252, 13.5344) (-30.4482, 13.5851) (-30.4715, 13.6356) (-30.4951, 13.6858) (-30.519, 13.7358) (-30.5432, 13.7855) (-30.5677, 13.835) (-30.5925, 13.8842) (-30.6176, 13.9331) (-30.643, 13.9817) (-30.6688, 14.0301) (-30.6948, 14.0782) (-30.7212, 14.126) (-30.7478, 14.1736) (-30.7748, 14.2208) (-30.8021, 14.2678) (-30.8297, 14.3144) (-30.8576, 14.3607) (-30.8859, 14.4067) (-30.9144, 14.4525) (-30.9433, 14.4978) (-30.9724, 14.5429) (-31.0019, 14.5876) (-31.0318, 14.632) (-31.0619, 14.6761) (-31.0924, 14.7198) (-31.1232, 14.7631) (-31.1543, 14.806) (-31.1858, 14.8486) (-31.2176, 14.8908) (-31.2497, 14.9327) (-31.2822, 14.9742) (-31.3149, 15.0152) (-31.3481, 15.0558) (-31.3816, 15.096) (-31.4155, 15.1356) (-31.4498, 15.1748) (-31.4844, 15.2136) (-31.5193, 15.2519) (-31.5546, 15.2898) (-31.5902, 15.3273) (-31.6262, 15.3643) (-31.6626, 15.4007) (-31.6995, 15.4364) (-31.7369, 15.4713) (-31.7748, 15.5054) (-31.8133, 15.5388) (-31.8521, 15.5716) (-31.8911, 15.6041) (-31.9305, 15.6361) (-31.9701, 15.6677) (-32.0103, 15.6982) (-32.0515, 15.7271) (-32.0855, 15.7484) (-32.1118, 15.763) (-32.1297, 15.7722) (-32.1388, 15.7767) knots -1 -1 -1 -1 -1 -1 -0.98571429 -0.97142857 -0.95714286 -0.94285714 -0.92857143 -0.91428571 -0.9 -0.88571429 -0.87142857 -0.85714286 -0.84285714 -0.82857143 -0.81428571 -0.8 -0.78571429 -0.77142857 -0.75714286 -0.74285714 -0.72857143 -0.71428571 -0.7 -0.68571429 -0.67142857 -0.65714286 -0.64285714 -0.62857143 -0.61428571 -0.6 -0.58571429 -0.57142857 -0.55714286 -0.54285714 -0.52857143 -0.51428571 -0.5 -0.48571429 -0.47142857 -0.45714286 -0.44285714 -0.42857143 -0.41428571 -0.4 -0.38571429 -0.37142857 -0.35714286 -0.34285714 -0.32857143 -0.31428571 -0.3 -0.28571429 -0.27142857 -0.25714286 -0.24285714 -0.22857143 -0.21428571 -0.2 -0.18571429 -0.17142857 -0.15714286 -0.14285714 -0.12857143 -0.11428571 -0.1 -0.08571429 -0.07142857 -0.05714286 -0.04285714 -0.02857143 -0.01428571 0 0 0 0 0 0
  line L9 (-32.1388, 15.7767) -> (-33.9159, 16.6494)
  arc A19 (-34.0653, 17.0651) -> (-33.9159, 16.6494) centre (-33.776, 16.9344) ccw
  arc A20 (-34.0653, 17.0651) -> (-33.4096, 19.0832) centre (-42.8517, 21.0355) ccw
  arc A21 (-33.0444, 19.3317) -> (-33.4096, 19.0832) centre (-33.0987, 19.0189) ccw
  line L10 (-33.0444, 19.3317) -> (-31.0937, 18.9932)
  spline S10 degree 5 poles (-31.0937, 18.9932) (-31.0837, 18.9915) (-31.0639, 18.9884) (-31.034, 18.9848) (-30.9939, 18.982) (-30.9436, 18.9811) (-30.8931, 18.9822) (-30.8425, 18.9844) (-30.7919, 18.9873) (-30.7412, 18.9905) (-30.6905, 18.9943) (-30.6398, 18.9987) (-30.5891, 19.004) (-30.5383, 19.0102) (-30.4874, 19.0174) (-30.4366, 19.0255) (-30.3858, 19.0343) (-30.3349, 19.0437) (-30.2841, 19.0536) (-30.2333, 19.0641) (-30.1825, 19.0751) (-30.1317, 19.0866) (-30.081, 19.0988) (-30.0303, 19.1116) (-29.9796, 19.125) (-29.9289, 19.1389) (-29.8783, 19.1534) (-29.8277, 19.1684) (-29.7772, 19.1838) (-29.7267, 19.1998) (-29.6763, 19.2162) (-29.6259, 19.2332) (-29.5756, 19.2506) (-29.5253, 19.2685) (-29.4751, 19.2869) (-29.4249, 19.3057) (-29.3748, 19.3251) (-29.3248, 19.3448) (-29.2748, 19.365) (-29.2249, 19.3857) (-29.1751, 19.4067) (-29.1254, 19.4282) (-29.0757, 19.4502) (-29.0261, 19.4725) (-28.9766, 19.4953) (-28.9272, 19.5185) (-28.8778, 19.5421) (-28.8286, 19.5661) (-28.7794, 19.5905) (-28.7303, 19.6154) (-28.6813, 19.6406) (-28.6324, 19.6662) (-28.5836, 19.6922) (-28.5349, 19.7185) (-28.4863, 19.7453) (-28.4378, 19.7724) (-28.3894, 19.8) (-28.3411, 19.8279) (-28.2929, 19.8561) (-28.2448, 19.8848) (-28.1968, 19.9138) (-28.1489, 19.9431) (-28.1012, 19.9728) (-28.0535, 20.0029) (-28.006, 20.0334) (-27.9586, 20.0642) (-27.9112, 20.0953) (-27.8641, 20.1268) (-27.817, 20.1586) (-27.7701, 20.1908) (-27.7232, 20.2233) (-27.6859, 20.2496) (-27.6579, 20.2695) (-27.6393, 20.2828) (-27.63, 20.2895) knots 0 0 0 0 0 0 0.01428571 0.02857143 0.04285714 0.05714286 0.07142857 0.08571429 0.1 0.11428571 0.12857143 0.14285714 0.15714286 0.17142857 0.18571429 0.2 0.21428571 0.22857143 0.24285714 0.25714286 0.27142857 0.28571429 0.3 0.31428571 0.32857143 0.34285714 0.35714286 0.37142857 0.38571429 0.4 0.41428571 0.42857143 0.44285714 0.45714286 0.47142857 0.48571429 0.5 0.51428571 0.52857143 0.54285714 0.55714286 0.57142857 0.58571429 0.6 0.61428571 0.62857143 0.64285714 0.65714286 0.67142857 0.68571429 0.7 0.71428571 0.72857143 0.74285714 0.75714286 0.77142857 0.78571429 0.8 0.81428571 0.82857143 0.84285714 0.85714286 0.87142857 0.88571429 0.9 0.91428571 0.92857143 0.94285714 0.95714286 0.97142857 0.98571429 1 1 1 1 1 1
  arc A22 (-27.63, 20.2895) -> (-27.63, 21.7816) centre (-42.8517, 21.0355) ccw
  spline S11 degree 5 poles (-27.63, 21.7816) (-27.6393, 21.7883) (-27.6579, 21.8016) (-27.6859, 21.8215) (-27.7232, 21.8478) (-27.7701, 21.8803) (-27.817, 21.9125) (-27.8641, 21.9443) (-27.9112, 21.9758) (-27.9586, 22.0069) (-28.006, 22.0377) (-28.0535, 22.0682) (-28.1012, 22.0982) (-28.1489, 22.128) (-28.1968, 22.1573) (-28.2448, 22.1863) (-28.2929, 22.215) (-28.3411, 22.2432) (-28.3894, 22.2711) (-28.4378, 22.2987) (-28.4863, 22.3258) (-28.5349, 22.3526) (-28.5836, 22.3789) (-28.6324, 22.4049) (-28.6813, 22.4305) (-28.7303, 22.4557) (-28.7794, 22.4806) (-28.8286, 22.505) (-28.8778, 22.529) (-28.9272, 22.5526) (-28.9766, 22.5758) (-29.0261, 22.5986) (-29.0757, 22.6209) (-29.1254, 22.6429) (-29.1751, 22.6644) (-29.2249, 22.6854) (-29.2748, 22.7061) (-29.3248, 22.7263) (-29.3748, 22.746) (-29.4249, 22.7653) (-29.4751, 22.7842) (-29.5253, 22.8026) (-29.5756, 22.8205) (-29.6259, 22.8379) (-29.6763, 22.8548) (-29.7267, 22.8713) (-29.7772, 22.8873) (-29.8277, 22.9027) (-29.8783, 22.9177) (-29.9289, 22.9322) (-29.9796, 22.9461) (-30.0303, 22.9595) (-30.081, 22.9723) (-30.1317, 22.9844) (-30.1825, 22.996) (-30.2333, 23.007) (-30.2841, 23.0175) (-30.3349, 23.0274) (-30.3858, 23.0368) (-30.4366, 23.0456) (-30.4874, 23.0537) (-30.5383, 23.0609) (-30.5891, 23.0671) (-30.6398, 23.0724) (-30.6905, 23.0768) (-30.7412, 23.0806) (-30.7919, 23.0838) (-30.8425, 23.0867) (-30.8931, 23.0889) (-30.9436, 23.09) (-30.9939, 23.0891) (-31.034, 23.0863) (-31.0639, 23.0827) (-31.0837, 23.0796) (-31.0937, 23.0779) knots -1 -1 -1 -1 -1 -1 -0.98571429 -0.97142857 -0.95714286 -0.94285714 -0.92857143 -0.91428571 -0.9 -0.88571429 -0.87142857 -0.85714286 -0.84285714 -0.82857143 -0.81428571 -0.8 -0.78571429 -0.77142857 -0.75714286 -0.74285714 -0.72857143 -0.71428571 -0.7 -0.68571429 -0.67142857 -0.65714286 -0.64285714 -0.62857143 -0.61428571 -0.6 -0.58571429 -0.57142857 -0.55714286 -0.54285714 -0.52857143 -0.51428571 -0.5 -0.48571429 -0.47142857 -0.45714286 -0.44285714 -0.42857143 -0.41428571 -0.4 -0.38571429 -0.37142857 -0.35714286 -0.34285714 -0.32857143 -0.31428571 -0.3 -0.28571429 -0.27142857 -0.25714286 -0.24285714 -0.22857143 -0.21428571 -0.2 -0.18571429 -0.17142857 -0.15714286 -0.14285714 -0.12857143 -0.11428571 -0.1 -0.08571429 -0.07142857 -0.05714286 -0.04285714 -0.02857143 -0.01428571 0 0 0 0 0 0
  line L11 (-31.0937, 23.0779) -> (-33.0444, 22.7394)
  arc A23 (-33.4096, 22.9879) -> (-33.0444, 22.7394) centre (-33.0987, 23.0522) ccw
  arc A24 (-33.4096, 22.9879) -> (-34.0653, 25.006) centre (-42.8517, 21.0355) ccw
  arc A25 (-33.9159, 25.4217) -> (-34.0653, 25.006) centre (-33.776, 25.1367) ccw
  line L12 (-33.9159, 25.4217) -> (-32.1388, 26.2944)
  spline S12 degree 5 poles (-32.1388, 26.2944) (-32.1297, 26.2989) (-32.1118, 26.308) (-32.0855, 26.3227) (-32.0515, 26.344) (-32.0103, 26.3729) (-31.9701, 26.4034) (-31.9305, 26.435) (-31.8911, 26.467) (-31.8521, 26.4994) (-31.8133, 26.5323) (-31.7748, 26.5657) (-31.7369, 26.5998) (-31.6995, 26.6347) (-31.6626, 26.6704) (-31.6262, 26.7068) (-31.5902, 26.7438) (-31.5546, 26.7812) (-31.5193, 26.8192) (-31.4844, 26.8575) (-31.4498, 26.8962) (-31.4155, 26.9355) (-31.3816, 26.9751) (-31.3481, 27.0153) (-31.3149, 27.0559) (-31.2822, 27.0969) (-31.2497, 27.1384) (-31.2176, 27.1803) (-31.1858, 27.2225) (-31.1543, 27.2651) (-31.1232, 27.308) (-31.0924, 27.3513) (-31.0619, 27.395) (-31.0318, 27.4391) (-31.0019, 27.4834) (-30.9724, 27.5282) (-30.9433, 27.5732) (-30.9144, 27.6186) (-30.8859, 27.6643) (-30.8576, 27.7104) (-30.8297, 27.7567) (-30.8021, 27.8033) (-30.7748, 27.8503) (-30.7478, 27.8975) (-30.7212, 27.945) (-30.6948, 27.9929) (-30.6688, 28.041) (-30.643, 28.0893) (-30.6176, 28.138) (-30.5925, 28.1869) (-30.5677, 28.2361) (-30.5432, 28.2856) (-30.519, 28.3353) (-30.4951, 28.3853) (-30.4715, 28.4355) (-30.4482, 28.486) (-30.4252, 28.5367) (-30.4025, 28.5876) (-30.3801, 28.6388) (-30.358, 28.6903) (-30.3363, 28.7419) (-30.3148, 28.7938) (-30.2936, 28.8459) (-30.2728, 28.8983) (-30.2522, 28.9509) (-30.2319, 29.0036) (-30.212, 29.0566) (-30.1923, 29.1099) (-30.1729, 29.1633) (-30.1539, 29.2169) (-30.1351, 29.2707) (-30.1203, 29.314) (-30.1094, 29.3465) (-30.1021, 29.3682) (-30.0985, 29.379) knots 0 0 0 0 0 0 0.01428571 0.02857143 0.04285714 0.05714286 0.07142857 0.08571429 0.1 0.11428571 0.12857143 0.14285714 0.15714286 0.17142857 0.18571429 0.2 0.21428571 0.22857143 0.24285714 0.25714286 0.27142857 0.28571429 0.3 0.31428571 0.32857143 0.34285714 0.35714286 0.37142857 0.38571429 0.4 0.41428571 0.42857143 0.44285714 0.45714286 0.47142857 0.48571429 0.5 0.51428571 0.52857143 0.54285714 0.55714286 0.57142857 0.58571429 0.6 0.61428571 0.62857143 0.64285714 0.65714286 0.67142857 0.68571429 0.7 0.71428571 0.72857143 0.74285714 0.75714286 0.77142857 0.78571429 0.8 0.81428571 0.82857143 0.84285714 0.85714286 0.87142857 0.88571429 0.9 0.91428571 0.92857143 0.94285714 0.95714286 0.97142857 0.98571429 1 1 1 1 1 1
  arc A26 (-30.0985, 29.379) -> (-30.9756, 30.5863) centre (-42.8517, 21.0355) ccw
  spline S13 degree 5 poles (-30.9756, 30.5863) (-30.9871, 30.5862) (-31.0099, 30.586) (-31.0443, 30.5857) (-31.0899, 30.585) (-31.1469, 30.5837) (-31.2038, 30.5822) (-31.2606, 30.5803) (-31.3173, 30.578) (-31.3739, 30.5754) (-31.4303, 30.5724) (-31.4867, 30.5691) (-31.5429, 30.5654) (-31.599, 30.5614) (-31.655, 30.557) (-31.7109, 30.5523) (-31.7666, 30.5472) (-31.8222, 30.5417) (-31.8777, 30.5359) (-31.933, 30.5297) (-31.9882, 30.5231) (-32.0433, 30.5162) (-32.0982, 30.5089) (-32.153, 30.5013) (-32.2076, 30.4933) (-32.262, 30.4849) (-32.3163, 30.4761) (-32.3705, 30.4669) (-32.4244, 30.4574) (-32.4782, 30.4475) (-32.5318, 30.4372) (-32.5853, 30.4265) (-32.6385, 30.4155) (-32.6916, 30.404) (-32.7445, 30.3922) (-32.7972, 30.38) (-32.8497, 30.3673) (-32.902, 30.3543) (-32.9541, 30.3409) (-33.0059, 30.3271) (-33.0576, 30.3128) (-33.109, 30.2982) (-33.1602, 30.2831) (-33.2112, 30.2676) (-33.2619, 30.2517) (-33.3124, 30.2354) (-33.3626, 30.2186) (-33.4126, 30.2014) (-33.4623, 30.1838) (-33.5118, 30.1658) (-33.561, 30.1473) (-33.6098, 30.1283) (-33.6584, 30.1088) (-33.7066, 30.0888) (-33.7545, 30.0684) (-33.802, 30.0474) (-33.8493, 30.026) (-33.8962, 30.0042) (-33.9429, 29.9819) (-33.9892, 29.9591) (-34.035, 29.9358) (-34.0804, 29.9117) (-34.1252, 29.8869) (-34.1693, 29.8614) (-34.2129, 29.8351) (-34.2562, 29.8084) (-34.2991, 29.7812) (-34.3417, 29.7538) (-34.3839, 29.7258) (-34.4254, 29.697) (-34.4656, 29.6668) (-34.4964, 29.6409) (-34.5185, 29.6205) (-34.5327, 29.6063) (-34.5397, 29.5991) knots -1 -1 -1 -1 -1 -1 -0.98571429 -0.97142857 -0.95714286 -0.94285714 -0.92857143 -0.91428571 -0.9 -0.88571429 -0.87142857 -0.85714286 -0.84285714 -0.82857143 -0.81428571 -0.8 -0.78571429 -0.77142857 -0.75714286 -0.74285714 -0.72857143 -0.71428571 -0.7 -0.68571429 -0.67142857 -0.65714286 -0.64285714 -0.62857143 -0.61428571 -0.6 -0.58571429 -0.57142857 -0.55714286 -0.54285714 -0.52857143 -0.51428571 -0.5 -0.48571429 -0.47142857 -0.45714286 -0.44285714 -0.42857143 -0.41428571 -0.4 -0.38571429 -0.37142857 -0.35714286 -0.34285714 -0.32857143 -0.31428571 -0.3 -0.28571429 -0.27142857 -0.25714286 -0.24285714 -0.22857143 -0.21428571 -0.2 -0.18571429 -0.17142857 -0.15714286 -0.14285714 -0.12857143 -0.11428571 -0.1 -0.08571429 -0.07142857 -0.05714286 -0.04285714 -0.02857143 -0.01428571 0 0 0 0 0 0
  line L13 (-34.5397, 29.5991) -> (-35.9189, 28.1786)
  arc A27 (-36.3604, 28.165) -> (-35.9189, 28.1786) centre (-36.1467, 28.3997) ccw
  arc A28 (-36.3604, 28.165) -> (-38.0771, 29.4122) centre (-42.8517, 21.0355) ccw
  arc A29 (-38.2006, 29.8364) -> (-38.0771, 29.4122) centre (-37.9199, 29.688) ccw
  line L14 (-38.2006, 29.8364) -> (-37.2759, 31.587)
  spline S14 degree 5 poles (-37.2759, 31.587) (-37.2712, 31.5959) (-37.2621, 31.6138) (-37.2494, 31.6411) (-37.2344, 31.6784) (-37.218, 31.726) (-37.2035, 31.7743) (-37.1899, 31.8231) (-37.177, 31.8722) (-37.1644, 31.9214) (-37.1523, 31.9707) (-37.1408, 32.0203) (-37.1302, 32.0702) (-37.1204, 32.1205) (-37.1116, 32.171) (-37.1035, 32.2218) (-37.0962, 32.2729) (-37.0894, 32.3242) (-37.0832, 32.3756) (-37.0774, 32.4271) (-37.0722, 32.4788) (-37.0675, 32.5307) (-37.0634, 32.5827) (-37.0599, 32.6349) (-37.0569, 32.6872) (-37.0545, 32.7397) (-37.0527, 32.7923) (-37.0513, 32.8451) (-37.0504, 32.8979) (-37.05, 32.9509) (-37.05, 33.0039) (-37.0506, 33.0571) (-37.0516, 33.1103) (-37.0531, 33.1637) (-37.055, 33.2171) (-37.0575, 33.2706) (-37.0603, 33.3243) (-37.0637, 33.3779) (-37.0674, 33.4317) (-37.0717, 33.4855) (-37.0763, 33.5394) (-37.0814, 33.5934) (-37.0869, 33.6474) (-37.0928, 33.7015) (-37.0992, 33.7556) (-37.106, 33.8098) (-37.1132, 33.864) (-37.1208, 33.9183) (-37.1288, 33.9726) (-37.1373, 34.0269) (-37.1461, 34.0813) (-37.1553, 34.1357) (-37.165, 34.1902) (-37.175, 34.2446) (-37.1855, 34.2991) (-37.1963, 34.3537) (-37.2075, 34.4082) (-37.2191, 34.4628) (-37.2311, 34.5173) (-37.2435, 34.5719) (-37.2562, 34.6265) (-37.2693, 34.6811) (-37.2828, 34.7357) (-37.2967, 34.7904) (-37.311, 34.845) (-37.3256, 34.8996) (-37.3406, 34.9542) (-37.356, 35.0088) (-37.3717, 35.0634) (-37.3878, 35.118) (-37.4043, 35.1726) (-37.4177, 35.2162) (-37.428, 35.249) (-37.4349, 35.2708) (-37.4383, 35.2817) knots 0 0 0 0 0 0 0.01428571 0.02857143 0.04285714 0.05714286 0.07142857 0.08571429 0.1 0.11428571 0.12857143 0.14285714 0.15714286 0.17142857 0.18571429 0.2 0.21428571 0.22857143 0.24285714 0.25714286 0.27142857 0.28571429 0.3 0.31428571 0.32857143 0.34285714 0.35714286 0.37142857 0.38571429 0.4 0.41428571 0.42857143 0.44285714 0.45714286 0.47142857 0.48571429 0.5 0.51428571 0.52857143 0.54285714 0.55714286 0.57142857 0.58571429 0.6 0.61428571 0.62857143 0.64285714 0.65714286 0.67142857 0.68571429 0.7 0.71428571 0.72857143 0.74285714 0.75714286 0.77142857 0.78571429 0.8 0.81428571 0.82857143 0.84285714 0.85714286 0.87142857 0.88571429 0.9 0.91428571 0.92857143 0.94285714 0.95714286 0.97142857 0.98571429 1 1 1 1 1 1
  arc A30 (-37.4383, 35.2817) -> (-38.8575, 35.7428) centre (-42.8517, 21.0355) ccw
  spline S15 degree 5 poles (-38.8575, 35.7428) (-38.8667, 35.736) (-38.8851, 35.7224) (-38.9127, 35.702) (-38.9492, 35.6746) (-38.9946, 35.6401) (-39.0397, 35.6054) (-39.0846, 35.5705) (-39.1291, 35.5353) (-39.1733, 35.4999) (-39.2173, 35.4644) (-39.2609, 35.4286) (-39.3042, 35.3925) (-39.3473, 35.3563) (-39.39, 35.3198) (-39.4324, 35.2832) (-39.4745, 35.2463) (-39.5163, 35.2092) (-39.5577, 35.1718) (-39.5988, 35.1343) (-39.6396, 35.0966) (-39.6801, 35.0586) (-39.7203, 35.0204) (-39.7601, 34.982) (-39.7995, 34.9435) (-39.8386, 34.9047) (-39.8774, 34.8656) (-39.9158, 34.8264) (-39.9539, 34.787) (-39.9916, 34.7474) (-40.0289, 34.7075) (-40.0659, 34.6675) (-40.1025, 34.6272) (-40.1387, 34.5868) (-40.1745, 34.5461) (-40.2099, 34.5052) (-40.245, 34.4641) (-40.2796, 34.4229) (-40.3139, 34.3814) (-40.3477, 34.3397) (-40.3812, 34.2978) (-40.4142, 34.2558) (-40.4467, 34.2135) (-40.4789, 34.171) (-40.5105, 34.1283) (-40.5418, 34.0854) (-40.5725, 34.0423) (-40.6029, 33.9991) (-40.6328, 33.9556) (-40.6622, 33.9119) (-40.6911, 33.868) (-40.7194, 33.824) (-40.7473, 33.7797) (-40.7745, 33.7352) (-40.8012, 33.6905) (-40.8274, 33.6456) (-40.853, 33.6005) (-40.8782, 33.5552) (-40.9029, 33.5098) (-40.9269, 33.4641) (-40.9503, 33.4183) (-40.9729, 33.3722) (-40.9945, 33.3258) (-41.0152, 33.2792) (-41.0351, 33.2323) (-41.0543, 33.1853) (-41.0731, 33.1381) (-41.0914, 33.0908) (-41.1091, 33.0433) (-41.1258, 32.9957) (-41.1405, 32.9476) (-41.1502, 32.9086) (-41.1561, 32.8791) (-41.1592, 32.8592) (-41.1607, 32.8492) knots -1 -1 -1 -1 -1 -1 -0.98571429 -0.97142857 -0.95714286 -0.94285714 -0.92857143 -0.91428571 -0.9 -0.88571429 -0.87142857 -0.85714286 -0.84285714 -0.82857143 -0.81428571 -0.8 -0.78571429 -0.77142857 -0.75714286 -0.74285714 -0.72857143 -0.71428571 -0.7 -0.68571429 -0.67142857 -0.65714286 -0.64285714 -0.62857143 -0.61428571 -0.6 -0.58571429 -0.57142857 -0.55714286 -0.54285714 -0.52857143 -0.51428571 -0.5 -0.48571429 -0.47142857 -0.45714286 -0.44285714 -0.42857143 -0.41428571 -0.4 -0.38571429 -0.37142857 -0.35714286 -0.34285714 -0.32857143 -0.31428571 -0.3 -0.28571429 -0.27142857 -0.25714286 -0.24285714 -0.22857143 -0.21428571 -0.2 -0.18571429 -0.17142857 -0.15714286 -0.14285714 -0.12857143 -0.11428571 -0.1 -0.08571429 -0.07142857 -0.05714286 -0.04285714 -0.02857143 -0.01428571 0 0 0 0 0 0
  line L15 (-41.1607, 32.8492) -> (-41.4415, 30.8894)
  arc A31 (-41.7907, 30.6188) -> (-41.4415, 30.8894) centre (-41.7558, 30.9344) ccw
  arc A32 (-41.7907, 30.6188) -> (-43.9127, 30.6188) centre (-42.8517, 21.0355) ccw
  arc A33 (-44.2619, 30.8894) -> (-43.9127, 30.6188) centre (-43.9476, 30.9344) ccw
  line L16 (-44.2619, 30.8894) -> (-44.5427, 32.8492)
  spline S16 degree 5 poles (-44.5427, 32.8492) (-44.5442, 32.8592) (-44.5473, 32.8791) (-44.5532, 32.9086) (-44.5629, 32.9476) (-44.5776, 32.9957) (-44.5943, 33.0433) (-44.612, 33.0908) (-44.6303, 33.1381) (-44.6491, 33.1853) (-44.6683, 33.2323) (-44.6882, 33.2792) (-44.7089, 33.3258) (-44.7305, 33.3722) (-44.7531, 33.4183) (-44.7765, 33.4641) (-44.8005, 33.5098) (-44.8252, 33.5552) (-44.8504, 33.6005) (-44.876, 33.6456) (-44.9022, 33.6905) (-44.9289, 33.7352) (-44.9561, 33.7797) (-44.984, 33.824) (-45.0123, 33.868) (-45.0412, 33.9119) (-45.0706, 33.9556) (-45.1005, 33.9991) (-45.1309, 34.0423) (-45.1616, 34.0854) (-45.1929, 34.1283) (-45.2245, 34.171) (-45.2567, 34.2135) (-45.2892, 34.2558) (-45.3222, 34.2978) (-45.3557, 34.3397) (-45.3895, 34.3814) (-45.4238, 34.4229) (-45.4584, 34.4641) (-45.4935, 34.5052) (-45.5289, 34.5461) (-45.5647, 34.5868) (-45.6009, 34.6272) (-45.6375, 34.6675) (-45.6745, 34.7075) (-45.7118, 34.7474) (-45.7495, 34.787) (-45.7876, 34.8264) (-45.826, 34.8656) (-45.8648, 34.9047) (-45.9039, 34.9435) (-45.9433, 34.982) (-45.9831, 35.0204) (-46.0233, 35.0586) (-46.0638, 35.0966) (-46.1046, 35.1343) (-46.1457, 35.1718) (-46.1871, 35.2092) (-46.2289, 35.2463) (-46.271, 35.2832) (-46.3134, 35.3198) (-46.3561, 35.3563) (-46.3992, 35.3925) (-46.4425, 35.4286) (-46.4861, 35.4644) (-46.5301, 35.4999) (-46.5743, 35.5353) (-46.6188, 35.5705) (-46.6637, 35.6054) (-46.7088, 35.6401) (-46.7542, 35.6746) (-46.7907, 35.702) (-46.8183, 35.7224) (-46.8367, 35.736) (-46.8459, 35.7428) knots 0 0 0 0 0 0 0.01428571 0.02857143 0.04285714 0.05714286 0.07142857 0.08571429 0.1 0.11428571 0.12857143 0.14285714 0.15714286 0.17142857 0.18571429 0.2 0.21428571 0.22857143 0.24285714 0.25714286 0.27142857 0.28571429 0.3 0.31428571 0.32857143 0.34285714 0.35714286 0.37142857 0.38571429 0.4 0.41428571 0.42857143 0.44285714 0.45714286 0.47142857 0.48571429 0.5 0.51428571 0.52857143 0.54285714 0.55714286 0.57142857 0.58571429 0.6 0.61428571 0.62857143 0.64285714 0.65714286 0.67142857 0.68571429 0.7 0.71428571 0.72857143 0.74285714 0.75714286 0.77142857 0.78571429 0.8 0.81428571 0.82857143 0.84285714 0.85714286 0.87142857 0.88571429 0.9 0.91428571 0.92857143 0.94285714 0.95714286 0.97142857 0.98571429 1 1 1 1 1 1
  arc A34 (-46.8459, 35.7428) -> (-48.2651, 35.2817) centre (-42.8517, 21.0355) ccw